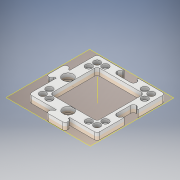
# Autodesk Inventor part: 10_Base_v2
Saved by Autodesk Inventor 2019 (Build 230136000, 136)
## iProperties
Created: 2017-06-20
Part Number: 10_Base_v2
Material: Generisch
Document SubType Name: Modeling
Designer: diederichbenedict
Density: 1 g/cm^3
Appearance: Weiß
Mass: 7.87446 g
Surface Area: 71.4468 cm^2
Volume: 7.87446 cm^3
d_part: 50,000 mm
d_o: 40,000 mm
d_i: 40,000 mm
Author: diederichbenedict
Autodesk Inventor part; units mm, degrees
ref_plane "YZ Plane" through (0, 0, 0) normal (1, 0, 0) x (0, 1, 0)
ref_plane "XZ Plane" through (0, 0, 0) normal (0, 1, 0) x (-1, 0, 0)
ref_plane "XY Plane" through (0, 0, 0) normal (0, 0, 1) x (1, 0, 0)
sketch "Skizze1" plane through (0, 0, 0) normal (0, 0, 1) x (1, 0, 0)
  line L0 (-17.95, -0.2) -> (-25.65, -0.2)
  line L1 (-25.65, -0.2) -> (-25.65, -23.2)
  line L2 (-23.65, -25.2) -> (-0.65, -25.2)
  line L3 (-0.65, -25.2) -> (-0.65, -17.5)
  line L4 (-17.95, -0.2) -> (-17.95, -15.5)
  line L5 (-15.95, -17.5) -> (-0.65, -17.5)
  arc A0 (-25.65, -23.2) -> (-23.65, -25.2) centre (-23.65, -23.2) ccw
  circle A1 centre (-20.55, -20.1) radius 2.4
  circle A2 centre (-21.2, -14.65) radius 2.45
  circle A3 centre (-15.1, -20.75) radius 2.45
  arc A4 (-17.95, -15.5) -> (-15.95, -17.5) centre (-15.95, -15.5) ccw
  circle A5 centre (-20.55, -20.1) radius 2.4
  circle A6 centre (-15.1, -20.75) radius 2.45
  point P0 (-25.65, -25.2)
  point P1 (-17.95, -17.5)
  dimension "d278" = 25
  dimension "d279" = 25
  dimension "d2" = 7.7
  dimension "d281" = 7.7
  dimension "d282" = 2
  dimension "d283" = 4.8
  dimension "d286" = 4.9
  dimension "d_hole" = 4.9
  dimension "d292" = 2
  dimension "d351" = 5.1
  dimension "d352" = 5.1
  dimension "d353" = 4.45
  dimension "d354" = 4.45
  dimension "d355" = 10.55
  dimension "d356" = 10.55
  constraints: 12 end point, 7 centre point, 4 point on circle, 4 point on line, 4 tangent, 2 coincident, 2 parallel, 1 horizontal, 1 perpendicular
  measures "d278" distance of L2.end point (-25.65, -25.2)
  measures "d279" distance of point (-25.65, -25.2) L0.end
  measures "d2" distance between parallel lines of L4 L1
  measures "d281" distance between parallel lines of L2 L5
  measures "d282" radius of A0
  measures "d283" diameter of A1
  measures "d286" diameter of A2
  measures "d_hole" diameter of A3
  measures "d292" radius of A4
  measures "d351" distance from line of L2 A1.centre
  measures "d352" distance from line of L1 A1.centre
  measures "d353" distance from line of L2 A3.centre
  measures "d354" distance from line of L1 A2.centre
  measures "d355" distance from line of L2 A2.centre
  measures "d356" distance from line of L1 A3.centre
extrude "Extrusion1" add sketch "Skizze1" along normal blind 5.1
mirror "Mirror6" about plane through (-17.95, -0.2, 0) normal (0, 1, 0) of "Extrusion1"
mirror "Mirror7" about plane through (-0.65, -25.2, 0) normal (1, 0, 0) of "Extrusion1", "Mirror6"
sketch "Sketch26" plane through (0, 0, 5.1) normal (0, 0, 1) x (1, 0, 0)
  line L0 (22.35, 24.8) -> (-23.65, 24.8) projected
  arc A0 (-23.65, 24.8) -> (-25.65, 22.8) centre (-23.65, 22.8) ccw projected
  line L1 (-25.65, -23.2) -> (-25.65, 22.8) projected
  arc A1 (-25.65, -23.2) -> (-23.65, -25.2) centre (-23.65, -23.2) ccw projected
  line L2 (-23.65, -25.2) -> (22.35, -25.2) projected
  arc A2 (22.35, -25.2) -> (24.35, -23.2) centre (22.35, -23.2) ccw projected
  line L3 (24.35, 22.8) -> (24.35, -23.2) projected
  arc A3 (24.35, 22.8) -> (22.35, 24.8) centre (22.35, 22.8) ccw projected
  line L4 (14.65, 17.1) -> (-15.95, 17.1) projected
  arc A4 (16.65, 15.1) -> (14.65, 17.1) centre (14.65, 15.1) ccw projected
  line L5 (16.65, 15.1) -> (16.65, -15.5) projected
  arc A5 (14.65, -17.5) -> (16.65, -15.5) centre (14.65, -15.5) ccw projected
  line L6 (-15.95, -17.5) -> (14.65, -17.5) projected
  arc A6 (-17.95, -15.5) -> (-15.95, -17.5) centre (-15.95, -15.5) ccw projected
  line L7 (-17.95, -15.5) -> (-17.95, 15.1) projected
  arc A7 (-15.95, 17.1) -> (-17.95, 15.1) centre (-15.95, 15.1) ccw projected
  line L8 (-25.65, -23.2) -> (-25.65, 22.8) projected
  line L9 (-28.9096, -7.14) -> (-29.05, -7.14)
  line L10 (-31.05, -5.14) -> (-31.05, -0.2)
  line L11 (-25.65, 6.8) -> (-25.65, -7.2)
  line L12 (-25.65, -5.2) -> (-26.4763, -5.2)
  line L13 (-26.9096, -5.2) -> (-25.5295, 4.7947) construction
  line L14 (-26.79, 4.8146) -> (-25.65, -5.2) construction
  line L15 (-26.9096, -5.2) -> (-26.9096, -5.14)
  line L16 (-26.79, 4.8146) -> (-26.79, 4.8146)
  arc A8 (-31.05, -5.14) -> (-29.05, -7.14) centre (-29.05, -5.14) ccw
  arc A9 (-28.9096, -7.14) -> (-26.95, -5.54) centre (-28.9096, -5.14) ccw
  arc A10 (-26.4763, -5.2) -> (-26.95, -5.54) centre (-26.4763, -5.7) ccw
  line L17 (-17.95, -15.5) -> (-17.95, 15.1) construction
  line L18 (-17.95, -0.2) -> (-38.1399, -0.2) construction
  line L19 (-26.95, -5.54) -> (-26.95, -0.2) construction
  line L20 (-28.9096, 6.74) -> (-29.05, 6.74)
  line L21 (-31.05, 4.74) -> (-31.05, -0.2)
  line L22 (-25.65, 4.8) -> (-26.4763, 4.8)
  arc A11 (-29.05, 6.74) -> (-31.05, 4.74) centre (-29.05, 4.74) ccw
  arc A12 (-26.95, 5.14) -> (-28.9096, 6.74) centre (-28.9096, 4.74) ccw
  arc A13 (-26.95, 5.14) -> (-26.4763, 4.8) centre (-26.4763, 5.3) ccw
  line L23 (-25.65, -5.2) -> (-25.65, 4.8)
  point P0 (0, 0)
  point P1 (-26.2192, -0.2)
  point P2 (-25.65, -0.2)
  dimension "d293" = 5.4
  dimension "d300" = 2
  dimension "d301" = 0.5
  dimension "d358" = 5
  dimension "d359" = 4.1
  dimension "d371" = 6.94
  constraints: 28 end point, 13 point on circle, 9 symmetric about line, 7 point on line, 6 centre point, 4 perpendicular, 4 tangent, 2 midpoint, 1 collinear, 1 equal radius, 1 horizontal, 1 parallel, 3 other
  measures "d293" distance between parallel lines of L1 L10
  measures "d300" radius of A8
  measures "d301" radius of A10
  measures "d358" distance between parallel lines of L18 L12
  measures "d359" distance between parallel lines of L19 L10
  measures "d371" distance between parallel lines of L18 L9
extrude "Extrusion13" add sketch "Sketch26" against normal up to surface (5.1 mm away) contours L1 L12 A10 A9 L9 A8 L10 L21 A11 L20 A12 A13 L22
sketch "Sketch27" plane through (0, 0, 5.1) normal (0, 0, 1) x (1, 0, 0)
  line L0 (22.35, 24.8) -> (-23.65, 24.8) projected
  arc A0 (-23.65, 24.8) -> (-25.65, 22.8) centre (-23.65, 22.8) ccw projected
  line L1 (-25.65, 4.8) -> (-25.65, 22.8) projected
  arc A1 (-25.65, -23.2) -> (-23.65, -25.2) centre (-23.65, -23.2) ccw projected
  line L2 (-23.65, -25.2) -> (22.35, -25.2) projected
  arc A2 (22.35, -25.2) -> (24.35, -23.2) centre (22.35, -23.2) ccw projected
  line L3 (24.35, 22.8) -> (24.35, -23.2) projected
  arc A3 (24.35, 22.8) -> (22.35, 24.8) centre (22.35, 22.8) ccw projected
  line L4 (14.65, 17.1) -> (-15.95, 17.1) projected
  arc A4 (16.65, 15.1) -> (14.65, 17.1) centre (14.65, 15.1) ccw projected
  line L5 (16.65, 15.1) -> (16.65, -15.5) projected
  arc A5 (14.65, -17.5) -> (16.65, -15.5) centre (14.65, -15.5) ccw projected
  line L6 (-15.95, -17.5) -> (14.65, -17.5) projected
  arc A6 (-17.95, -15.5) -> (-15.95, -17.5) centre (-15.95, -15.5) ccw projected
  line L7 (-17.95, -15.5) -> (-17.95, 15.1) projected
  arc A7 (-15.95, 17.1) -> (-17.95, 15.1) centre (-15.95, 15.1) ccw projected
  circle A8 centre (-0.65, -0.2) radius 17.3
  line L8 (-25.65, 4.8) -> (-26.4763, 4.8) projected
  arc A9 (-26.95, 5.14) -> (-26.4763, 4.8) centre (-26.4763, 5.3) ccw projected
  arc A10 (-26.95, 5.14) -> (-28.9096, 6.74) centre (-28.9096, 4.74) ccw projected
  line L9 (-28.9096, 6.74) -> (-29.05, 6.74) projected
  arc A11 (-29.05, 6.74) -> (-31.05, 4.74) centre (-29.05, 4.74) ccw projected
  line L10 (-31.05, 4.74) -> (-31.05, -5.14) projected
  arc A12 (-31.05, -5.14) -> (-29.05, -7.14) centre (-29.05, -5.14) ccw projected
  line L11 (-29.05, -7.14) -> (-28.9096, -7.14) projected
  arc A13 (-28.9096, -7.14) -> (-26.95, -5.54) centre (-28.9096, -5.14) ccw projected
  arc A14 (-26.4763, -5.2) -> (-26.95, -5.54) centre (-26.4763, -5.7) ccw projected
  line L12 (-26.4763, -5.2) -> (-25.65, -5.2) projected
  line L13 (-25.65, -23.2) -> (-25.65, -5.2) projected
  point P0 (0, 0)
  constraints: 3 tangent, 1 centre point
sketch "Sketch28" plane through (0, 0, 5.1) normal (0, 0, 1) x (1, 0, 0)
  line L0 (22.35, 24.8) -> (-23.65, 24.8) projected
  arc A0 (-23.65, 24.8) -> (-25.65, 22.8) centre (-23.65, 22.8) ccw projected
  line L1 (-25.65, 4.8) -> (-25.65, 22.8) projected
  arc A1 (-25.65, -23.2) -> (-23.65, -25.2) centre (-23.65, -23.2) ccw projected
  line L2 (-23.65, -25.2) -> (22.35, -25.2) projected
  arc A2 (22.35, -25.2) -> (24.35, -23.2) centre (22.35, -23.2) ccw projected
  line L3 (24.35, 22.8) -> (24.35, -23.2) projected
  arc A3 (24.35, 22.8) -> (22.35, 24.8) centre (22.35, 22.8) ccw projected
  line L4 (14.65, 17.1) -> (-15.95, 17.1) projected
  arc A4 (16.65, 15.1) -> (14.65, 17.1) centre (14.65, 15.1) ccw projected
  line L5 (16.65, 15.1) -> (16.65, -15.5) projected
  arc A5 (14.65, -17.5) -> (16.65, -15.5) centre (14.65, -15.5) ccw projected
  line L6 (-15.95, -17.5) -> (14.65, -17.5) projected
  arc A6 (-17.95, -15.5) -> (-15.95, -17.5) centre (-15.95, -15.5) ccw projected
  line L7 (-17.95, -15.5) -> (-17.95, 15.1) projected
  arc A7 (-15.95, 17.1) -> (-17.95, 15.1) centre (-15.95, 15.1) ccw projected
  line L8 (-25.65, 22.8) -> (-25.65, -23.2) projected
  line L9 (-25.65, 4.8) -> (-26.4763, 4.8) projected
  arc A8 (-26.95, 5.14) -> (-26.4763, 4.8) centre (-26.4763, 5.3) ccw projected
  arc A9 (-26.95, 5.14) -> (-28.9096, 6.74) centre (-28.9096, 4.74) ccw projected
  line L10 (-28.9096, 6.74) -> (-29.05, 6.74) projected
  arc A10 (-29.05, 6.74) -> (-31.05, 4.74) centre (-29.05, 4.74) ccw projected
  line L11 (-31.05, 4.74) -> (-31.05, -5.14) projected
  arc A11 (-31.05, -5.14) -> (-29.05, -7.14) centre (-29.05, -5.14) ccw projected
  line L12 (-29.05, -7.14) -> (-28.9096, -7.14) projected
  arc A12 (-28.9096, -7.14) -> (-26.95, -5.54) centre (-28.9096, -5.14) ccw projected
  arc A13 (-26.4763, -5.2) -> (-26.95, -5.54) centre (-26.4763, -5.7) ccw projected
  line L13 (-26.4763, -5.2) -> (-25.65, -5.2) projected
  line L14 (-25.65, -23.2) -> (-25.65, -5.2) projected
  arc A14 (-31.05, -5.14) -> (-29.05, -7.14) centre (-29.05, -5.14) ccw projected
  line L15 (-31.05, -5.14) -> (-31.05, 4.74)
  arc A15 (-29.05, 6.74) -> (-31.05, 4.74) centre (-29.05, 4.74) ccw projected
  line L16 (-29.05, 6.74) -> (-28.9096, 6.74)
  line L17 (-25.65, 4.8) -> (-26.4763, 4.8) projected
  line L18 (-26.4763, 4.8) -> (-25.65, 4.8)
  line L19 (-25.65, 4.8) -> (-25.65, -5.2)
  arc A16 (-28.9096, -7.14) -> (-26.95, -5.54) centre (-28.9096, -5.14) ccw projected
  line L20 (-28.9096, -7.14) -> (-29.05, -7.14)
  arc A17 (-31.05, -5.14) -> (-29.05, -7.14) centre (-29.05, -5.14) ccw
  arc A18 (-28.9096, -7.14) -> (-26.95, -5.54) centre (-28.9096, -5.14) ccw
  arc A19 (-26.4763, -5.2) -> (-26.95, -5.54) centre (-26.4763, -5.7) ccw projected
  arc A20 (-26.4763, -5.2) -> (-26.95, -5.54) centre (-26.4763, -5.7) ccw
  arc A21 (-26.95, 5.14) -> (-26.4763, 4.8) centre (-26.4763, 5.3) ccw projected
  arc A22 (-26.95, 5.14) -> (-26.4763, 4.8) centre (-26.4763, 5.3) ccw
  arc A23 (-29.05, 6.74) -> (-31.05, 4.74) centre (-29.05, 4.74) ccw
  line L21 (-25.65, -5.2) -> (-26.4763, -5.2) projected
  line L22 (-26.4763, -5.2) -> (-25.65, -5.2)
  line L23 (-31.05, 4.74) -> (-31.05, -5.14) construction
  arc A24 (-26.95, 5.14) -> (-28.9096, 6.74) centre (-28.9096, 4.74) ccw projected
  arc A25 (-26.95, 5.14) -> (-28.9096, 6.74) centre (-28.9096, 4.74) ccw
  line L24 (-31.25, 4.74) -> (-31.25, -5.14)
  arc A26 (-31.25, -5.14) -> (-29.05, -7.34) centre (-29.05, -5.14) ccw
  line L25 (-29.05, -7.34) -> (-28.9096, -7.34)
  arc A27 (-28.9096, -7.34) -> (-26.757, -5.594) centre (-28.9096, -5.14) ccw
  arc A28 (-26.4763, -5.4) -> (-26.757, -5.594) centre (-26.4763, -5.7) ccw
  line L26 (-26.4763, -5.4) -> (-25.45, -5.4)
  line L27 (-25.45, -5.4) -> (-25.45, 5)
  line L28 (-25.45, 5) -> (-26.4763, 5)
  arc A29 (-26.757, 5.194) -> (-26.4763, 5) centre (-26.4763, 5.3) ccw
  arc A30 (-26.757, 5.194) -> (-28.9096, 6.94) centre (-28.9096, 4.74) ccw
  line L29 (-28.9096, 6.94) -> (-29.05, 6.94)
  arc A31 (-29.05, 6.94) -> (-31.25, 4.74) centre (-29.05, 4.74) ccw
  line L30 (24.35, 22.8) -> (24.35, -23.2) construction
  line L31 (24.35, -0.2) -> (-31.05, -0.2) construction
  line L32 (24.35, 6.75) -> (18.85, 6.75) construction
  line L33 (18.85, 6.75) -> (18.85, -7.15) construction
  line L34 (18.85, -7.15) -> (24.35, -7.15) construction
  line L35 (24.35, -7.15) -> (24.35, 6.75) construction
  line L36 (24.35, 6.75) -> (18.85, -7.15) construction
  line L37 (18.85, 6.75) -> (24.35, -7.15) construction
  line L38 (18.9998, -5.1434) -> (19.0003, 4.7402)
  line L39 (21.0504, 6.79) -> (21.1908, 6.79)
  line L40 (23.624, 4.8502) -> (24.4489, 4.8503)
  line L41 (24.4489, 4.8503) -> (24.4489, -5.2511)
  line L42 (21.1907, -7.1947) -> (21.0509, -7.1947)
  arc A32 (18.9998, -5.1434) -> (21.0509, -7.1947) centre (21.0509, -5.1435) ccw
  arc A33 (21.1907, -7.1947) -> (23.2033, -5.5537) centre (21.1907, -5.14) ccw
  arc A34 (23.6238, -5.2509) -> (23.2033, -5.5537) centre (23.6278, -5.6999) ccw
  arc A35 (23.1986, 5.153) -> (23.624, 4.8502) centre (23.6239, 5.3004) ccw
  arc A36 (21.0504, 6.79) -> (19.0003, 4.7402) centre (21.0503, 4.74) ccw
  line L43 (23.6238, -5.2509) -> (24.4489, -5.2511)
  arc A37 (23.1986, 5.153) -> (21.1908, 6.79) centre (21.1906, 4.7401) ccw
  line L44 (18.9003, 4.74) -> (18.8998, -5.1434)
  arc A38 (18.8998, -5.1434) -> (21.0509, -7.2947) centre (21.0509, -5.1435) ccw
  line L45 (21.0509, -7.2947) -> (21.1907, -7.2947)
  arc A39 (21.1907, -7.2947) -> (23.2998, -5.5806) centre (21.1907, -5.14) ccw
  arc A40 (23.6242, -5.3509) -> (23.2998, -5.5806) centre (23.6278, -5.6999) ccw
  line L46 (23.6242, -5.3509) -> (24.5489, -5.3512)
  line L47 (24.5489, -5.3512) -> (24.5489, 4.9503)
  line L48 (24.5489, 4.9503) -> (23.6239, 4.9502)
  arc A41 (23.2951, 5.18) -> (23.6239, 4.9502) centre (23.6239, 5.3004) ccw
  arc A42 (23.2951, 5.18) -> (21.1907, 6.89) centre (21.1906, 4.7401) ccw
  line L49 (21.1907, 6.89) -> (21.0504, 6.89)
  arc A43 (21.0504, 6.89) -> (18.9003, 4.74) centre (21.0503, 4.74) ccw
  point P0 (0, 0)
  point P1 (21.6, -0.2)
  point P2 (19.0503, -0.2)
  dimension "d372" = 0.2
  dimension "d373" = 2.2
  dimension "d374" = 13.9
  dimension "d375" = 0.1
  constraints: 62 end point, 49 point on circle, 24 centre point, 12 tangent, 9 perpendicular, 5 collinear, 4 midpoint, 2 parallel, 1 horizontal, 1 point on line, 22 other
  measures "d372" radial gap between concentric circles of A23 A31
  measures "d373" distance between parallel lines of L5 L33
  measures "d374" distance between parallel lines of L32 L34
  measures "d375" radial gap between concentric circles of A36 A43
extrude "Extrusion14" cut sketch "Sketch28" against normal blind 10 contours L48 L47 L46 L3 L43 L41 L40 | L3 L40 A35 A37 L39 A36 L38 A32 L42 A33 A34 L43 L46 A40 A39 L45 A38 L44 A43 L49 A42 A41 L48 | L40 L41 L43 L3 | L3 L43 A34 A33 L42 A32 L38 A36 L39 A37 A35 L40
pattern_circular "Circular Pattern6" count 2 over 90 about axis through (-0.65, -0.2, 5.1) along (0, 0, 1) of "Extrusion14", "Extrusion13"
sketch "Sketch29" plane through (0, 0, 5.1) normal (0, 0, 1) x (1, 0, 0)
  line L0 (-5.8002, 24.8) -> (-23.65, 24.8) projected
  arc A0 (-23.65, 24.8) -> (-25.65, 22.8) centre (-23.65, 22.8) ccw projected
  line L1 (-25.65, 4.8) -> (-25.65, 22.8) projected
  arc A1 (-25.65, -23.2) -> (-23.65, -25.2) centre (-23.65, -23.2) ccw projected
  line L2 (-23.65, -25.2) -> (-5.65, -25.2) projected
  arc A2 (22.35, -25.2) -> (24.35, -23.2) centre (22.35, -23.2) ccw projected
  line L3 (24.35, -5.3511) -> (24.35, -23.2) projected
  arc A3 (24.35, 22.8) -> (22.35, 24.8) centre (22.35, 22.8) ccw projected
  line L4 (14.65, 17.1) -> (-15.95, 17.1) projected
  arc A4 (16.65, 15.1) -> (14.65, 17.1) centre (14.65, 15.1) ccw projected
  line L5 (16.65, 15.1) -> (16.65, -15.5) projected
  arc A5 (14.65, -17.5) -> (16.65, -15.5) centre (14.65, -15.5) ccw projected
  line L6 (-15.95, -17.5) -> (14.65, -17.5) projected
  arc A6 (-17.95, -15.5) -> (-15.95, -17.5) centre (-15.95, -15.5) ccw projected
  line L7 (-17.95, -15.5) -> (-17.95, 15.1) projected
  arc A7 (-15.95, 17.1) -> (-17.95, 15.1) centre (-15.95, 15.1) ccw projected
  circle A8 centre (-21.95, -0.3) radius 3.89
  circle A9 centre (-0.55, -21.5) radius 2.9259
  line L8 (-25.65, 4.8) -> (-26.4763, 4.8) projected
  arc A10 (-26.95, 5.14) -> (-26.4763, 4.8) centre (-26.4763, 5.3) ccw projected
  arc A11 (-26.95, 5.14) -> (-28.9096, 6.74) centre (-28.9096, 4.74) ccw projected
  line L9 (-28.9096, 6.74) -> (-29.05, 6.74) projected
  arc A12 (-29.05, 6.74) -> (-31.05, 4.74) centre (-29.05, 4.74) ccw projected
  line L10 (-31.05, 4.74) -> (-31.05, -5.14) projected
  arc A13 (-31.05, -5.14) -> (-29.05, -7.14) centre (-29.05, -5.14) ccw projected
  line L11 (-29.05, -7.14) -> (-28.9096, -7.14) projected
  arc A14 (-28.9096, -7.14) -> (-26.95, -5.54) centre (-28.9096, -5.14) ccw projected
  arc A15 (-26.4763, -5.2) -> (-26.95, -5.54) centre (-26.4763, -5.7) ccw projected
  line L12 (-26.4763, -5.2) -> (-25.65, -5.2) projected
  line L13 (-25.65, -23.2) -> (-25.65, -5.2) projected
  line L14 (-5.65, -25.2) -> (-5.65, -26.0263) projected
  arc A16 (-5.99, -26.5) -> (-5.65, -26.0263) centre (-6.15, -26.0263) ccw projected
  arc A17 (-5.99, -26.5) -> (-7.59, -28.4596) centre (-5.59, -28.4596) ccw projected
  line L15 (-7.59, -28.4596) -> (-7.59, -28.6) projected
  arc A18 (-7.59, -28.6) -> (-5.59, -30.6) centre (-5.59, -28.6) ccw projected
  line L16 (-5.59, -30.6) -> (4.29, -30.6) projected
  arc A19 (4.29, -30.6) -> (6.29, -28.6) centre (4.29, -28.6) ccw projected
  line L17 (6.29, -28.6) -> (6.29, -28.4596) projected
  arc A20 (6.29, -28.4596) -> (4.69, -26.5) centre (4.29, -28.4596) ccw projected
  arc A21 (4.35, -26.0263) -> (4.69, -26.5) centre (4.85, -26.0263) ccw projected
  line L18 (4.35, -26.0263) -> (4.35, -25.2) projected
  line L19 (4.35, -25.2) -> (22.35, -25.2) projected
  line L20 (4.5011, 24.8) -> (4.5009, 24.0742) projected
  arc A22 (4.5009, 24.0742) -> (4.7306, 23.7498) centre (4.8499, 24.0778) ccw projected
  arc A23 (6.4447, 21.6407) -> (4.7306, 23.7498) centre (4.29, 21.6407) ccw projected
  line L21 (6.4447, 21.6407) -> (6.4447, 21.5009) projected
  arc A24 (4.2934, 19.3498) -> (6.4447, 21.5009) centre (4.2935, 21.5009) ccw projected
  line L22 (4.2934, 19.3498) -> (-5.59, 19.3503) projected
  arc A25 (-7.74, 21.5004) -> (-5.59, 19.3503) centre (-5.59, 21.5003) ccw projected
  line L23 (-7.74, 21.5004) -> (-7.74, 21.6407) projected
  arc A26 (-6.03, 23.7451) -> (-7.74, 21.6407) centre (-5.5901, 21.6406) ccw projected
  arc A27 (-6.03, 23.7451) -> (-5.8002, 24.0739) centre (-6.1504, 24.0739) ccw projected
  line L24 (-5.8002, 24.0739) -> (-5.8002, 24.8) projected
  line L25 (24.35, -5.3511) -> (23.6242, -5.3509) projected
  arc A28 (23.6242, -5.3509) -> (23.2998, -5.5806) centre (23.6278, -5.6999) ccw projected
  arc A29 (21.1907, -7.2947) -> (23.2998, -5.5806) centre (21.1907, -5.14) ccw projected
  line L26 (21.1907, -7.2947) -> (21.0509, -7.2947) projected
  arc A30 (18.8998, -5.1434) -> (21.0509, -7.2947) centre (21.0509, -5.1435) ccw projected
  line L27 (18.8998, -5.1434) -> (18.9003, 4.74) projected
  arc A31 (21.0504, 6.89) -> (18.9003, 4.74) centre (21.0503, 4.74) ccw projected
  line L28 (21.0504, 6.89) -> (21.1907, 6.89) projected
  arc A32 (23.2951, 5.18) -> (21.1907, 6.89) centre (21.1906, 4.7401) ccw projected
  arc A33 (23.2951, 5.18) -> (23.6239, 4.9502) centre (23.6239, 5.3004) ccw projected
  line L29 (23.6239, 4.9502) -> (24.35, 4.9502) projected
  line L30 (24.35, 22.8) -> (24.35, 4.9502) projected
  line L31 (22.35, 24.8) -> (4.5011, 24.8) projected
  point P0 (0, 0)
  dimension "d319" = 7.78
  dimension "d320" = 4
  dimension "d321" = 21.4
  dimension "d322" = 4
  constraints: 2 centre point, 1 coincident
  measures "d319" diameter of A8
  measures "d320" distance from line of A8.centre L7
  measures "d321" horizontal distance of A9.centre A8.centre
  measures "d322" distance from line of L6 A9.centre
hole "Hole7" at (-21.95, -0.3, 5.1) at (-0.55, -21.5, 5.1) direction (0, 0, -1) diameter 4.3 end through all counterbore diameter 7.8 counterbore depth 4
pattern_circular "Circular Pattern7" count 2 over 90 about axis through (-0.65, -0.2, 5.1) along (0, 0, 1) of "Extrusion14", "Extrusion13"
ref_plane "Work Plane14" through (0, 0, 2.55) normal (0, 0, 1) x (1, 0, 0)
sketch "Sketch32" plane through (0, 0, 2.55) normal (0, 0, 1) x (1, 0, 0)
  circle A0 centre (-21.2, -14.65) radius 2.45 projected
  circle A1 centre (-15.1, -20.75) radius 2.45 projected
  circle A2 centre (13.8, -20.75) radius 2.45 projected
  circle A3 centre (19.9, -14.65) radius 2.45 projected
  circle A4 centre (19.9, 14.25) radius 2.45 projected
  circle A5 centre (13.8, 20.35) radius 2.45 projected
  circle A6 centre (-15.1, 20.35) radius 2.45 projected
  circle A7 centre (-21.2, 14.25) radius 2.45 projected
  point P0 (0, 0)
extrude "Extrusion16" add sketch "Sketch32" along normal mid plane 0.3
equation "\"d_i\" = 40"
equation "\"d_o\" = 40"
equation "\"d_part\" = 50"
equation "\"d6\" = 0"
equation "\"d7\" = 0"
equation "\"d8\" = 0"
equation "\"d9\" = 0"
equation "\"d13\" = 0"
equation "\"d14\" = 0"
equation "\"d20\" = 0"
equation "\"d21\" = 0"
equation "\"d22\" = 0"
equation "\"d23\" = 0"
equation "\"d24\" = 0"
equation "\"d25\" = 3"
equation "\"d26\" = 0"
equation "\"d27\" = 0"
equation "\"d28\" = 0"
equation "\"d29\" = 0"
equation "\"d30\" = 0"
equation "\"d31\" = 0"
equation "\"d32\" = 0"
equation "\"d33\" = 0"
equation "\"d34\" = 0"
equation "\"d46\" = 0"
equation "\"d47\" = 0"
equation "\"d48\" = 0"
equation "\"d50\" = 0"
equation "\"d51\" = 0"
equation "\"d52\" = 0"
equation "\"d53\" = 0"
equation "\"d54\" = 0"
equation "\"d55\" = 0"
equation "\"d56\" = 0"
equation "\"d57\" = 0"
equation "\"d58\" = 0"
equation "\"d59\" = 0"
equation "\"magnet_offset\" = 0"
equation "\"screw_offset\" = 0"
equation "\"mal_puzzle_offset\" = 0"
equation "\"fem_puzzle_offset\" = 0"
